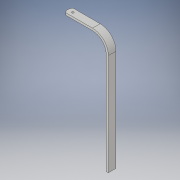
# Autodesk Inventor part: topbar
Saved by Autodesk Inventor 2019.3 (Build 233278000, 278)
## iProperties
Created: 2019-04-14
Part Number: topbar
Material: Generic
Document SubType Name: Modeling
Designer: peter
Density: 1 g/cm^3
Appearance: Default
Author: peter
Autodesk Inventor part; units mm, degrees
ref_plane "YZ Plane" through (0, 0, 0) normal (1, 0, 0) x (0, 1, 0)
ref_plane "XZ Plane" through (0, 0, 0) normal (0, 1, 0) x (-1, 0, 0)
ref_plane "XY Plane" through (0, 0, 0) normal (0, 0, 1) x (1, 0, 0)
sketch "Sketch1" plane through (0, 0, 0) normal (0, 0, 1) x (1, 0, 0)
  line L0 (0, 0) -> (45, 0)
  line L1 (45, 0) -> (45, 0)
  line L2 (70, -25) -> (70, -25)
  line L3 (70, -25) -> (70, -185)
  arc A0 (70, -25) -> (45, 0) centre (45, -25) ccw
  arc A1 (66.5, -25) -> (45, -3.5) centre (45, -25) ccw
  line L4 (45, -3.5) -> (0, -3.5)
  line L5 (0, -3.5) -> (0, 0)
  line L6 (66.5, -25) -> (66.5, -185)
  line L7 (66.5, -25) -> (226.5, -25) construction
  line L8 (66.5, -185) -> (70, -185)
  point P0 (70, 0)
  dimension "d0" = 45
  dimension "d1" = 25
  dimension "d2" = 25
  dimension "d3" = 160
  dimension "d4" = 25
  dimension "d5" = 43
  dimension "d6" = 160
  dimension "d7" = 90
  constraints: 18 end point, 4 point on circle, 4 point on line, 3 horizontal, 3 perpendicular, 2 centre point, 2 tangent, 1 coincident, 1 parallel, 1 vertical
  measures "d0" distance of L0.start L0.end
  measures "d1" distance of L0.end point (70, 0)
  measures "d2" distance of point (70, 0) L2.end
  measures "d3" distance of L2.end L3.end
  measures "d4" radius of A0
  measures "d5" diameter of A1
  measures "d6" distance of L6.start L6.end
  measures "d7" angle of L6 L7
extrude "Extrusion1" add sketch "Sketch1" along normal blind 12
sketch "Sketch2" plane through (0, 0, 0) normal (0, 1, 0) x (1, 0, 0)
  line L0 (0, 0) -> (0, -12) construction
  line L1 (0, -6) -> (8, -6) construction
  circle A0 centre (8, -6) radius 1.5
  line L2 (0, 0) -> (2, 0) construction
  line L3 (2, 0) -> (2, -12) construction
  line L4 (45, -12) -> (0, -12) construction
  line L5 (2, -12) -> (0, -12) construction
  arc A1 (2.7085, 0) -> (2.7085, -12) centre (8, -6) ccw
  line L6 (0, 0) -> (45, 0) projected
  line L7 (0, 0) -> (0, -12) projected
  line L8 (45, -12) -> (0, -12) projected
  line L9 (45, 0) -> (45, -12) projected
  dimension "d10" = 8
  dimension "d11" = 3
  dimension "d12" = 2
  constraints: 8 end point, 3 point on circle, 2 centre point, 2 coincident, 2 horizontal, 2 perpendicular, 2 point on line, 1 midpoint
  measures "d10" distance of L1.start L1.end
  measures "d11" diameter of A0
  measures "d12" distance of L0.start L2.end
extrude "Extrusion2" cut sketch "Sketch2" along normal through all both and the other way through all contours A0 | A1 L7 L6 | A1 L8 L7
body "Solid1"
